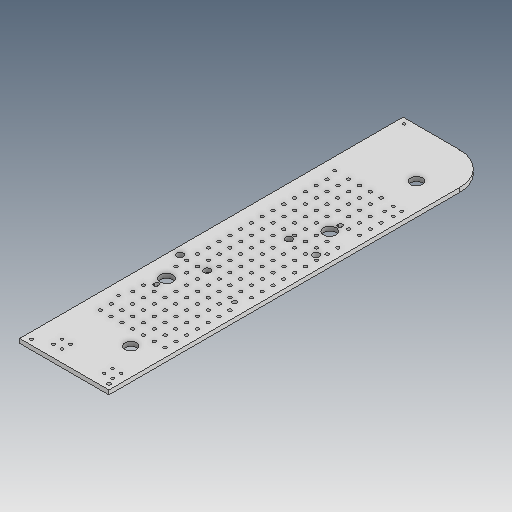
# Autodesk Inventor part: sidewall inside
Saved by Autodesk Inventor 2020 (Build 240168000, 168)
## iProperties
Created: 2020-03-01
Part Number: sidewall inside
Material: Generic
Document SubType Name: Modeling
Designer: ball
Density: 1 g/cm^3
Appearance: Default
Author: ball
Autodesk Inventor part; units mm, degrees
ref_plane "YZ Plane" through (0, 0, 0) normal (1, 0, 0) x (0, 1, 0)
ref_plane "XZ Plane" through (0, 0, 0) normal (0, 1, 0) x (-1, 0, 0)
ref_plane "XY Plane" through (0, 0, 0) normal (0, 0, 1) x (1, 0, 0)
sketch "Sketch1" plane through (0, 0, 0) normal (0, 1, 0) x (-1, 0, 0)
  line L0 (0, 0) -> (104.9602, 0)
  line L1 (104.9602, 0) -> (104.9602, -450.85)
  line L2 (104.9602, -450.85) -> (38.1, -450.85)
  line L3 (0, -412.75) -> (0, 0)
  arc A0 (0, -412.75) -> (38.1, -450.85) centre (38.1, -412.75) ccw
  line L4 (38.1, -412.75) -> (38.1, -450.85) construction
  line L5 (38.1, -412.75) -> (76.2, -412.75) construction
  dimension "d1" = 450.85
  dimension "d5" = 38.1
  dimension "d6" = 90
  dimension "d7" = 104.9602
  dimension "d8" = 38.1
  constraints: 12 end point, 2 horizontal, 2 parallel, 2 perpendicular, 2 point on circle, 1 centre point, 1 coincident
  measures "d1" distance of L0.end L1.end
  measures "d5" radius of A0
  measures "d6" angle of L4 L5
  measures "d7" distance between parallel lines of L3 L1
  measures "d8" distance from line of L3 point (38.1, -412.75)
extrude "Extrusion1" add sketch "Sketch1" along normal blind 5
sketch "Sketch2" plane through (0, 5, 0) normal (0, 1, 0) x (1, 0, 0)
  circle A0 centre (-31.75, 57.3786) radius 6.95
  line L0 (-104.9602, 0) -> (0, 0) projected
  line L1 (0, 0) -> (0, 412.75) projected
  circle A1 centre (-31.75, 393.4714) radius 6.95
  circle A2 centre (-9.8044, 14.0462) radius 1.65
  circle A3 centre (-9.8044, 24.0462) radius 1.65
  circle A4 centre (-19.8044, 14.0462) radius 1.65
  circle A5 centre (-19.8044, 24.0462) radius 1.65
  circle A6 centre (-69.342, 14.0462) radius 1.65
  circle A7 centre (-79.342, 14.0462) radius 1.65
  circle A8 centre (-69.342, 24.0462) radius 1.65
  circle A9 centre (-79.342, 24.0462) radius 1.65
  circle A10 centre (-10.16, 76.2) radius 1.905
  circle A11 centre (-10.16, 88.9) radius 1.905
  circle A12 centre (-10.16, 101.6) radius 1.905
  circle A13 centre (-10.16, 114.3) radius 1.905
  circle A14 centre (-10.16, 127) radius 1.905
  circle A15 centre (-10.16, 139.7) radius 1.905
  circle A16 centre (-10.16, 152.4) radius 1.905
  circle A17 centre (-10.16, 165.1) radius 1.905
  circle A18 centre (-10.16, 177.8) radius 1.905
  circle A19 centre (-10.16, 190.5) radius 1.905
  circle A20 centre (-10.16, 203.2) radius 1.905
  circle A21 centre (-10.16, 215.9) radius 1.905
  circle A22 centre (-10.16, 228.6) radius 1.905
  circle A23 centre (-10.16, 241.3) radius 1.905
  circle A24 centre (-10.16, 254) radius 1.905
  circle A25 centre (-10.16, 266.7) radius 1.905
  circle A26 centre (-10.16, 279.4) radius 1.905
  circle A27 centre (-10.16, 292.1) radius 1.905
  circle A28 centre (-10.16, 304.8) radius 1.905
  circle A29 centre (-10.16, 317.5) radius 1.905
  circle A30 centre (-10.16, 330.2) radius 1.905
  circle A31 centre (-10.16, 342.9) radius 1.905
  circle A32 centre (-10.16, 355.6) radius 1.905
  circle A33 centre (-22.86, 76.2) radius 1.905
  circle A34 centre (-22.86, 88.9) radius 1.905
  circle A35 centre (-22.86, 101.6) radius 1.905
  circle A36 centre (-22.86, 114.3) radius 1.905
  circle A37 centre (-22.86, 127) radius 1.905
  circle A38 centre (-22.86, 139.7) radius 1.905
  circle A39 centre (-22.86, 152.4) radius 1.905
  circle A40 centre (-22.86, 165.1) radius 1.905
  circle A41 centre (-22.86, 177.8) radius 1.905
  circle A42 centre (-22.86, 190.5) radius 1.905
  circle A43 centre (-22.86, 203.2) radius 1.905
  circle A44 centre (-22.86, 215.9) radius 1.905
  circle A45 centre (-22.86, 228.6) radius 1.905
  circle A46 centre (-22.86, 241.3) radius 1.905
  circle A47 centre (-22.86, 254) radius 1.905
  circle A48 centre (-22.86, 266.7) radius 1.905
  circle A49 centre (-22.86, 279.4) radius 1.905
  circle A50 centre (-22.86, 292.1) radius 1.905
  circle A51 centre (-22.86, 304.8) radius 1.905
  circle A52 centre (-22.86, 317.5) radius 1.905
  circle A53 centre (-22.86, 330.2) radius 1.905
  circle A54 centre (-22.86, 342.9) radius 1.905
  circle A55 centre (-22.86, 355.6) radius 1.905
  circle A56 centre (-35.56, 76.2) radius 1.905
  circle A57 centre (-35.56, 88.9) radius 1.905
  circle A58 centre (-35.56, 101.6) radius 1.905
  circle A59 centre (-35.56, 114.3) radius 1.905
  circle A60 centre (-35.56, 127) radius 1.905
  circle A61 centre (-35.56, 139.7) radius 1.905
  circle A62 centre (-35.56, 152.4) radius 1.905
  circle A63 centre (-35.56, 165.1) radius 1.905
  circle A64 centre (-35.56, 177.8) radius 1.905
  circle A65 centre (-35.56, 190.5) radius 1.905
  circle A66 centre (-35.56, 203.2) radius 1.905
  circle A67 centre (-35.56, 215.9) radius 1.905
  circle A68 centre (-35.56, 228.6) radius 1.905
  circle A69 centre (-35.56, 241.3) radius 1.905
  circle A70 centre (-35.56, 254) radius 1.905
  circle A71 centre (-35.56, 266.7) radius 1.905
  circle A72 centre (-35.56, 279.4) radius 1.905
  circle A73 centre (-35.56, 292.1) radius 1.905
  circle A74 centre (-35.56, 304.8) radius 1.905
  circle A75 centre (-35.56, 317.5) radius 1.905
  circle A76 centre (-35.56, 330.2) radius 1.905
  circle A77 centre (-35.56, 342.9) radius 1.905
  circle A78 centre (-35.56, 355.6) radius 1.905
  circle A79 centre (-48.26, 76.2) radius 1.905
  circle A80 centre (-48.26, 88.9) radius 1.905
  circle A81 centre (-48.26, 101.6) radius 1.905
  circle A82 centre (-48.26, 114.3) radius 1.905
  circle A83 centre (-48.26, 127) radius 1.905
  circle A84 centre (-48.26, 139.7) radius 1.905
  circle A85 centre (-48.26, 152.4) radius 1.905
  circle A86 centre (-48.26, 165.1) radius 1.905
  circle A87 centre (-48.26, 177.8) radius 1.905
  circle A88 centre (-48.26, 190.5) radius 1.905
  circle A89 centre (-48.26, 203.2) radius 1.905
  circle A90 centre (-48.26, 215.9) radius 1.905
  circle A91 centre (-48.26, 228.6) radius 1.905
  circle A92 centre (-48.26, 241.3) radius 1.905
  circle A93 centre (-48.26, 254) radius 1.905
  circle A94 centre (-48.26, 266.7) radius 1.905
  circle A95 centre (-48.26, 279.4) radius 1.905
  circle A96 centre (-48.26, 292.1) radius 1.905
  circle A97 centre (-48.26, 304.8) radius 1.905
  circle A98 centre (-48.26, 317.5) radius 1.905
  circle A99 centre (-48.26, 330.2) radius 1.905
  circle A100 centre (-48.26, 342.9) radius 1.905
  circle A101 centre (-48.26, 355.6) radius 1.905
  circle A102 centre (-60.96, 76.2) radius 1.905
  circle A103 centre (-60.96, 88.9) radius 1.905
  circle A104 centre (-60.96, 101.6) radius 1.905
  circle A105 centre (-60.96, 114.3) radius 1.905
  circle A106 centre (-60.96, 127) radius 1.905
  circle A107 centre (-60.96, 139.7) radius 1.905
  circle A108 centre (-60.96, 152.4) radius 1.905
  circle A109 centre (-60.96, 165.1) radius 1.905
  circle A110 centre (-60.96, 177.8) radius 1.905
  circle A111 centre (-60.96, 190.5) radius 1.905
  circle A112 centre (-60.96, 203.2) radius 1.905
  circle A113 centre (-60.96, 215.9) radius 1.905
  circle A114 centre (-60.96, 228.6) radius 1.905
  circle A115 centre (-60.96, 241.3) radius 1.905
  circle A116 centre (-60.96, 254) radius 1.905
  circle A117 centre (-60.96, 266.7) radius 1.905
  circle A118 centre (-60.96, 279.4) radius 1.905
  circle A119 centre (-60.96, 292.1) radius 1.905
  circle A120 centre (-60.96, 304.8) radius 1.905
  circle A121 centre (-60.96, 317.5) radius 1.905
  circle A122 centre (-60.96, 330.2) radius 1.905
  circle A123 centre (-60.96, 342.9) radius 1.905
  circle A124 centre (-60.96, 355.6) radius 1.905
  circle A125 centre (-73.66, 76.2) radius 1.905
  circle A126 centre (-73.66, 88.9) radius 1.905
  circle A127 centre (-73.66, 101.6) radius 1.905
  circle A128 centre (-73.66, 114.3) radius 1.905
  circle A129 centre (-73.66, 127) radius 1.905
  circle A130 centre (-73.66, 139.7) radius 1.905
  circle A131 centre (-73.66, 152.4) radius 1.905
  circle A132 centre (-73.66, 165.1) radius 1.905
  circle A133 centre (-73.66, 177.8) radius 1.905
  circle A134 centre (-73.66, 190.5) radius 1.905
  circle A135 centre (-73.66, 203.2) radius 1.905
  circle A136 centre (-73.66, 215.9) radius 1.905
  circle A137 centre (-73.66, 228.6) radius 1.905
  circle A138 centre (-73.66, 241.3) radius 1.905
  circle A139 centre (-73.66, 254) radius 1.905
  circle A140 centre (-73.66, 266.7) radius 1.905
  circle A141 centre (-73.66, 279.4) radius 1.905
  circle A142 centre (-73.66, 292.1) radius 1.905
  circle A143 centre (-73.66, 304.8) radius 1.905
  circle A144 centre (-73.66, 317.5) radius 1.905
  circle A145 centre (-73.66, 330.2) radius 1.905
  circle A146 centre (-73.66, 342.9) radius 1.905
  circle A147 centre (-73.66, 355.6) radius 1.905
  circle A148 centre (-86.36, 76.2) radius 1.905
  circle A149 centre (-86.36, 88.9) radius 1.905
  circle A150 centre (-86.36, 101.6) radius 1.905
  circle A151 centre (-86.36, 114.3) radius 1.905
  circle A152 centre (-86.36, 127) radius 1.905
  circle A153 centre (-86.36, 139.7) radius 1.905
  circle A154 centre (-86.36, 152.4) radius 1.905
  circle A155 centre (-86.36, 165.1) radius 1.905
  circle A156 centre (-86.36, 177.8) radius 1.905
  circle A157 centre (-86.36, 190.5) radius 1.905
  circle A158 centre (-86.36, 203.2) radius 1.905
  circle A159 centre (-86.36, 215.9) radius 1.905
  circle A160 centre (-86.36, 228.6) radius 1.905
  circle A161 centre (-86.36, 241.3) radius 1.905
  circle A162 centre (-86.36, 254) radius 1.905
  circle A163 centre (-86.36, 266.7) radius 1.905
  circle A164 centre (-86.36, 279.4) radius 1.905
  circle A165 centre (-86.36, 292.1) radius 1.905
  circle A166 centre (-86.36, 304.8) radius 1.905
  circle A167 centre (-86.36, 317.5) radius 1.905
  circle A168 centre (-86.36, 330.2) radius 1.905
  circle A169 centre (-86.36, 342.9) radius 1.905
  circle A170 centre (-86.36, 355.6) radius 1.905
  circle A171 centre (-9.8044, 344.2462) radius 1.65
  circle A172 centre (-9.8044, 354.2462) radius 1.65
  circle A173 centre (-19.8044, 344.2462) radius 1.65
  circle A174 centre (-19.8044, 354.2462) radius 1.65
  circle A175 centre (-6.35, 6.35) radius 2.15
  line L2 (-19.8044, 24.0462) -> (-9.8044, 14.0462) construction
  line L3 (-9.8044, 24.0462) -> (-19.8044, 14.0462) construction
  line L4 (-22.3044, 26.5462) -> (-7.3044, 26.5462) construction
  line L5 (-7.3044, 26.5462) -> (-7.3044, 11.5462) construction
  line L6 (-7.3044, 11.5462) -> (-22.3044, 11.5462) construction
  line L7 (-22.3044, 11.5462) -> (-22.3044, 26.5462) construction
  line L8 (-22.3044, 26.5462) -> (-7.3044, 11.5462) construction
  line L9 (-7.3044, 26.5462) -> (-22.3044, 11.5462) construction
  point P0 (-14.8044, 19.0462)
  dimension "BearingHole" = 13.9
  dimension "d12" = 57.3786
  dimension "d13" = 31.75
  dimension "d14" = 13.9
  dimension "d15" = 31.75
  dimension "d16" = 336.0928
  dimension "M3Clearance" = 3.3
  dimension "d20" = 14.0462
  dimension "d21" = 9.8044
  dimension "d24" = 10
  dimension "d27" = 10
  dimension "d30" = 3.3
  dimension "d31" = 14.0462
  dimension "d32" = 69.342
  dimension "d42" = 10
  dimension "d45" = 10
  dimension "Number6Clearance" = 3.81
  dimension "d49" = 10.16
  dimension "d50" = 76.2
  dimension "d53" = 12.7
  dimension "d56" = 12.7
  dimension "d59" = 3.3
  dimension "d60" = 9.8044
  dimension "d61" = 344.2462
  dimension "d64" = 10
  dimension "d67" = 10
  dimension "M4Clearance" = 4.3
  dimension "d71" = 6.35
  dimension "d72" = 6.35
  dimension "d73" = 15
  dimension "d74" = 15
  constraints: 176 centre point, 16 end point, 5 horizontal, 4 vertical, 3 midpoint, 2 parallel, 1 perpendicular, 338 other
  measures "BearingHole" diameter of A0
  measures "d12" distance from line of L0 A0.centre
  measures "d13" distance from line of L1 A0.centre
  measures "d14" diameter of A1
  measures "d15" distance from line of L1 A1.centre
  measures "d16" distance of A0.centre A1.centre
  measures "M3Clearance" diameter of A2
  measures "d20" distance from line of L0 L2.end
  measures "d21" distance from line of L1 L2.end
  measures "d24" distance of L2.end L3.start
  measures "d27" distance of L2.end L3.end
  measures "d30" diameter of A6
  measures "d31" distance from line of L0 A6.centre
  measures "d32" distance from line of L1 A6.centre
  measures "d42" distance of A6.centre A7.centre
  measures "d45" distance of A6.centre A8.centre
  measures "Number6Clearance" diameter of A10
  measures "d49" distance from line of L1 A10.centre
  measures "d50" distance from line of L0 A10.centre
  measures "d53" distance of A10.centre A11.centre
  measures "d56" distance of A10.centre A33.centre
  measures "d59" diameter of A171
  measures "d60" distance from line of L1 A171.centre
  measures "d61" distance from line of L0 A171.centre
  measures "d64" distance of A171.centre A172.centre
  measures "d67" distance of A171.centre A173.centre
  measures "M4Clearance" diameter of A175
  measures "d71" distance from line of L1 A175.centre
  measures "d72" distance from line of L0 A175.centre
  measures "d73" distance of L5.end L6.end
  measures "d74" distance of L4.end L5.end
extrude "Extrusion2" cut sketch "Sketch2" against normal through all contours A0 | A1 | A2 | A3 | A4 | A5 | A6 | A7 | A8 | A9 | A10 | A11 | A12 | A13 | A14 | A15 | A16 | A18 | A19 | A20 | A21 | A22 | A23 | A24 | A25 | A26 | A28 | A29 | A30 | A171 A31 | A31 A171 | A172 A32 | A32 A172 | A33 | A34 | A35 | A36 | A37 | A38 | A39 | A40 | A41 | A42 | A43 | A44 | A45 | A46 | A47 | A48 | A49 | A51 | A52 | A53 | A173 A54 | A54 A173 | A174 A55 | A55 A174 | A56 | A57 | A58 | A59 | A60 | A61 | A62 | A63 | A64 | A65 | A66 | A67 | A68 | A69 | A70 | A71 | A72 | A73 | A75 | A76 | A77 | A78 | A79 | A80 | A81 | A82 | A83 | A84 | A85 | A86 | A87 | A88 | A89 | A90 | A91 | A92 | A94 | A95 | A96 | A97 | A98 | A99 | A100 | A101 | A102 | A103 | A104 | A105 | A106 | A107 | A108 | A109 | A111 | A112 | A113 | A114 | A115 | A116 | A117 | A118 | A119 | A120 | A121 | A122 | A123 | A124 | A125 | A126 | A127 | A128 | A129 | A132 | A133 | A134 | A135 | A136 | A137 | A138 | A139 | A140 | A141 | A142 | A143 | A144 | A145 | A146 | A147 | A148 | A149 | A151 | A152 | A155 | A156 | A157 | A158 | A159 | A160 | A161 | A162 | A163 | A164 | A165 | A166 | A167 | A168 | A169 | A175 picked at (-9.7937, 344.0241) picked at (-9.5179, 345.0808) picked at (-9.7948, 354.473) picked at (-9.5205, 353.4158) picked at (-21.1894, 343.636) picked at (-20.2006, 344.1162) picked at (-21.2712, 354.8215) picked at (-20.2017, 354.3785)
sketch "Sketch3" plane through (0, 5, 0) normal (0, 1, 0) x (1, 0, 0)
  circle A0 centre (-97.3271, 444.4951) radius 1.7 construction
  circle A1 centre (-97.3271, 6.3451) radius 1.7 construction
  circle A2 centre (-63.6771, 179.4247) radius 3.15 construction
  circle A3 centre (-95.6771, 179.4247) radius 3.5 construction
  circle A4 centre (-79.6771, 147.4247) radius 7 construction
  circle A5 centre (-31.6771, 291.4247) radius 7 construction
  circle A6 centre (-15.6771, 259.4247) radius 3.5 construction
  circle A7 centre (-47.6771, 259.4247) radius 3.5 construction
  circle A8 centre (-31.75, 393.4714) radius 6.95 construction
  circle A9 centre (-15.6771, 163.4247) radius 2.25 construction
  arc A10 (-33.6771, 302.7384) -> (-29.6771, 302.7384) centre (-31.6771, 302.7384) ccw construction
  arc A11 (-29.6771, 304.111) -> (-33.6771, 304.111) centre (-31.6771, 304.111) ccw construction
  line L0 (-29.6771, 302.7384) -> (-29.6771, 304.111) construction
  line L1 (-33.6771, 304.111) -> (-33.6771, 302.7384) construction
  line L2 (-77.6771, 158.7384) -> (-77.6771, 160.111) construction
  arc A12 (-77.6771, 160.111) -> (-81.6771, 160.111) centre (-79.6771, 160.111) ccw construction
  line L3 (-81.6771, 160.111) -> (-81.6771, 158.7384) construction
  arc A13 (-81.6771, 158.7384) -> (-77.6771, 158.7384) centre (-79.6771, 158.7384) ccw construction
  circle A14 centre (-97.3271, 6.3451) radius 1.65
  circle A15 centre (-97.3271, 444.4951) radius 1.65
  circle A16 centre (-79.6771, 147.4247) radius 7.5
  circle A17 centre (-31.6771, 291.4247) radius 7.5
  circle A18 centre (-95.6771, 179.4247) radius 4
  circle A19 centre (-63.6771, 179.4247) radius 4
  circle A20 centre (-15.6771, 259.4247) radius 4
  circle A21 centre (-47.6771, 259.4247) radius 4
  circle A22 centre (-15.6771, 163.4247) radius 2.413
  arc A23 (-77.6771, 136.111) -> (-81.6771, 136.111) centre (-79.6771, 136.111) ccw construction
  line L4 (-77.6771, 134.7384) -> (-77.6771, 136.111) construction
  line L5 (-81.6771, 136.111) -> (-81.6771, 134.7384) construction
  arc A24 (-81.6771, 134.7384) -> (-77.6771, 134.7384) centre (-79.6771, 134.7384) ccw construction
  circle A25 centre (-90.4602, 355.95) radius 1.7 construction
  circle A26 centre (-90.4602, 355.95) radius 1.65
  circle A27 centre (-90.4602, 101.631) radius 1.7 construction
  circle A28 centre (-90.4602, 101.631) radius 1.65
  arc A29 (-77.3108, 136.111) -> (-82.0433, 136.111) centre (-79.6771, 136.111) ccw
  line L6 (-77.3108, 136.111) -> (-77.3108, 134.7384)
  arc A30 (-82.0433, 134.7384) -> (-77.3108, 134.7384) centre (-79.6771, 134.7384) ccw
  line L7 (-82.0433, 134.7384) -> (-82.0433, 136.111)
  arc A31 (-29.4142, 304.111) -> (-33.9399, 304.111) centre (-31.6771, 304.111) ccw
  line L8 (-29.4142, 304.111) -> (-29.4142, 302.7384)
  arc A32 (-33.9399, 302.7384) -> (-29.4142, 302.7384) centre (-31.6771, 302.7384) ccw
  line L9 (-33.9399, 302.7384) -> (-33.9399, 304.111)
  point P0 (0, 0)
  dimension "d75" = 3.3
  dimension "d76" = 3.3
  dimension "BearingClearance" = 15
  dimension "d78" = 15
  dimension "M4HeadClearance" = 8
  dimension "d80" = 8
  dimension "d81" = 8
  dimension "d82" = 8
  dimension "d83" = 4.826
  dimension "d90" = 3.3
  dimension "d91" = 3.3
  dimension "d92" = 0.3663
  dimension "d93" = 0.2628
  constraints: 15 centre point, 11 coincident, 8 end point, 8 point on circle, 6 other
  measures "d75" diameter of A14
  measures "d76" diameter of A15
  measures "BearingClearance" diameter of A16
  measures "d78" diameter of A17
  measures "M4HeadClearance" diameter of A18
  measures "d80" diameter of A19
  measures "d81" diameter of A20
  measures "d82" diameter of A21
  measures "d83" diameter of A22
  measures "d90" diameter of A26
  measures "d91" diameter of A28
  measures "d92" radial gap between concentric circles of A23 A29
  measures "d93" radial gap between concentric circles of A11 A31
extrude "Extrusion3" cut sketch "Sketch3" against normal through all
equation "\"d14\" = BearingHole"
equation "\"d15\" = d13"
equation "\"d30\" = M3Clearance"
equation "\"d31\" = d20"
equation "\"d59\" = M3Clearance"
equation "\"d60\" = d21"
equation "\"d75\" = M3Clearance"
equation "\"d76\" = M3Clearance"
equation "\"d78\" = BearingClearance"
equation "\"d80\" = M4HeadClearance"
equation "\"d81\" = M4HeadClearance"
equation "\"d82\" = M4HeadClearance"
equation "\"d90\" = M3Clearance"
equation "\"d91\" = M3Clearance"
body "Solid1"
